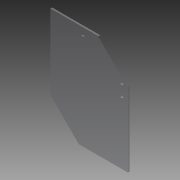
# Autodesk Inventor part: Wireless Mounting Board
Saved by Autodesk Inventor 2014 SP1 (Build 180222100, 222)
## iProperties
Created: 2013-10-26
Part Number: Wireless Mounting Board
Material: Polycarbonate, Clear
Document SubType Name: Modeling
Designer: Moses
Mass: 117.44 g
Surface Area: 641.762 cm^2
Volume: 97.8671 cm^3
Density: 1.2 g/cm^3
Appearance: Polycarbonate - Clear
Author: Moses
Autodesk Inventor part; units mm, degrees
ref_plane "YZ Plane" through (0, 0, 0) normal (1, 0, 0) x (0, 1, 0)
ref_plane "XZ Plane" through (0, 0, 0) normal (0, 1, 0) x (-1, 0, 0)
ref_plane "XY Plane" through (0, 0, 0) normal (0, 0, 1) x (1, 0, 0)
sketch "Sketch1" plane through (0, 0, 0) normal (0, 0, 1) x (1, 0, 0)
  line L0 (0, 0) -> (152.4, 0)
  line L1 (152.4, 0) -> (152.4, 203.2)
  line L2 (152.4, 203.2) -> (0, 203.2)
  line L3 (0, 203.2) -> (0, 0)
  circle A0 centre (63.5, 190.5) radius 3.3782 projected
  circle A1 centre (139.7, 146.05) radius 3.3782 projected
  circle A2 centre (139.7, 123.825) radius 3.3782 projected
  circle A3 centre (114.3, 190.5) radius 3.3782 projected
  dimension "d0" = 152.4
  dimension "d1" = 203.2
  constraints: 8 end point, 2 parallel, 1 horizontal, 1 perpendicular
  measures "d0" distance of L1.end L2.end
  measures "d1" distance of L0.end L1.end
extrude "Extrusion1" add sketch "Sketch1" along normal blind 3.175
body "Solid1"
